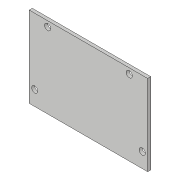
# Autodesk Inventor part: Sensor Case Lid
Saved by Autodesk Inventor 2018.3 (Build 223284000, 284)
## iProperties
Created: 2019-04-12
Part Number: Sensor Case Lid
Material: Generic
Document SubType Name: Modeling
Designer: aye06091
Mass: 3.91466 g
Surface Area: 53.1837 cm^2
Volume: 3.91466 cm^3
Density: 1 g/cm^3
Appearance: Default
Author: aye06091
Autodesk Inventor part; units mm, degrees
ref_plane "YZ Plane" through (0, 0, 0) normal (1, 0, 0) x (0, 1, 0)
ref_plane "XZ Plane" through (0, 0, 0) normal (0, 1, 0) x (-1, 0, 0)
ref_plane "XY Plane" through (0, 0, 0) normal (0, 0, 1) x (1, 0, 0)
sketch "Sketch1" plane through (0, 0, 0) normal (0, 0, 1) x (1, 0, 0)
  line L0 (0, 0) -> (60.5112, 0)
  line L1 (60.5112, 0) -> (60.5112, -41.275)
  line L2 (60.5112, -41.275) -> (0, -41.275)
  line L3 (0, -41.275) -> (0, 0)
  dimension "d0" = 41.275
  dimension "d1" = 60.5112
  constraints: 8 end point, 2 parallel, 1 horizontal, 1 perpendicular
  measures "d0" distance of L2.end L0.start
  measures "d1" distance of L0.start L0.end
extrude "Extrusion1" add sketch "Sketch1" against normal blind 1.5875
sketch "Sketch2" plane through (0, 0, 0) normal (0, 0, 1) x (1, 0, 0)
  line L0 (0, 0) -> (60.5112, 0) projected
  line L1 (0, -41.275) -> (0, 0) projected
  line L2 (60.5112, -41.275) -> (0, -41.275) projected
  line L3 (60.5112, 0) -> (60.5112, -41.275) projected
  circle A0 centre (2.8067, -33.7185) radius 1.5875
  circle A1 centre (57.7045, -33.7185) radius 1.5875
  circle A2 centre (9.4234, -2.8067) radius 1.5875
  circle A3 centre (51.0878, -2.8067) radius 1.5875
  dimension "d13" = 3.175
  dimension "d14" = 2.8067
  dimension "d15" = 7.5565
  dimension "d16" = 3.175
  dimension "d17" = 7.5565
  dimension "d18" = 2.8067
  dimension "d19" = 3.175
  dimension "d20" = 9.4234
  dimension "d21" = 9.4234
  dimension "d22" = 3.175
  dimension "d23" = 2.8067
  dimension "d24" = 2.8067
  constraints: 4 centre point
  measures "d13" diameter of A0
  measures "d14" distance from line of L1 A0.centre
  measures "d15" distance from line of L2 A0.centre
  measures "d16" diameter of A1
  measures "d17" distance from line of L2 A1.centre
  measures "d18" distance from line of L3 A1.centre
  measures "d19" diameter of A2
  measures "d20" distance from line of L1 A2.centre
  measures "d21" distance from line of L3 A3.centre
  measures "d22" diameter of A3
  measures "d23" distance from line of L0 A3.centre
  measures "d24" distance from line of L0 A2.centre
extrude "Extrusion2" cut sketch "Sketch2" against normal blind 1.5875 contours A0 | A1 | A2 | A3
body "Solid1"
